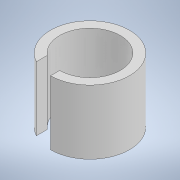
# Autodesk Inventor part: BearingTest
Saved by Autodesk Inventor 2022 (Build 260153000, 153)
## iProperties
Created: 2022-04-15
Part Number: BearingTest
Material: Generic
Document SubType Name: Modeling
Designer: awp
Density: 1 g/cm^3
Appearance: Default
Author: awp
Autodesk Inventor part; units mm, degrees
ref_plane "YZ Plane" through (0, 0, 0) normal (1, 0, 0) x (0, 1, 0)
ref_plane "XZ Plane" through (0, 0, 0) normal (0, 1, 0) x (-1, 0, 0)
ref_plane "XY Plane" through (0, 0, 0) normal (0, 0, 1) x (1, 0, 0)
sketch "Sketch1" plane through (0, 0, 0) normal (0, 1, 0) x (-1, 0, 0)
  circle A0 centre (0, 0) radius 3
  circle A1 centre (0, 0) radius 3.9
  line L0 (-0.9525, -4.3342) -> (0.9525, -4.3342)
  line L1 (0.9525, -4.3342) -> (0.9525, 4.3342)
  line L2 (0.9525, 4.3342) -> (-0.9525, 4.3342)
  line L3 (-0.9525, 4.3342) -> (-0.9525, -4.3342)
  line L4 (-0.9525, -4.3342) -> (0.9525, 4.3342) construction
  line L5 (0.9525, -4.3342) -> (-0.9525, 4.3342) construction
  line L6 (0, 0) -> (1.905, 0)
  line L7 (1.905, 0) -> (1.905, 6.1107)
  line L8 (1.905, 6.1107) -> (0, 6.1107)
  line L9 (0, 6.1107) -> (0, 0)
  point P0 (-0.9525, 2.8448)
  point P1 (-0.9525, 3.7819)
  point P2 (0.9525, 3.7819)
  point P3 (0.9525, 2.8448)
  point P4 (1.905, 3.4031)
  point P5 (1.905, 2.3175)
  point P6 (0, 3)
  point P7 (0, 3.9)
  dimension "d0" = 6
  dimension "d1" = 7.8
  dimension "d4" = 1.905
  dimension "d5" = 1.905
  constraints: 20 end point, 4 parallel, 2 centre point, 2 coincident, 2 horizontal, 2 midpoint, 2 perpendicular
  measures "d0" diameter of A0
  measures "d1" diameter of A1
  measures "d4" distance of L0.start L0.end
  measures "d5" distance of L8.end L7.end
extrude "Extrusion1" add sketch "Sketch1" along normal blind 6.35 contours A0 L7 A1 L1 | L1 A1 L3 A0 | L3 A1 A0 | A0 L3 A1 L9 picked at (3.5685, -0.2846)
body "Solid1"
